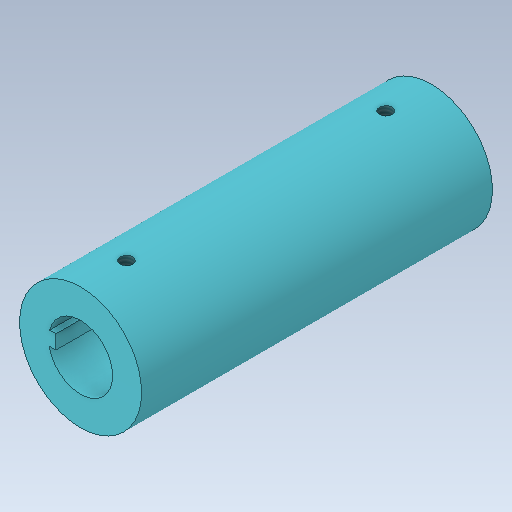
# Autodesk Inventor part: ShaftToConnectPotToMotor
Saved by Autodesk Inventor 2020.1 (Build 241239000, 239)
## iProperties
Created: 2018-02-27
Part Number: ShaftToConnectPotToMotor
Material: Aluminum 6061
Document SubType Name: Modeling
Designer: steele
Density: 2.7 g/cm^3
Appearance: Cadet Blue
Author: steele
Autodesk Inventor part; units mm, degrees
ref_plane "YZ Plane" through (0, 0, 0) normal (1, 0, 0) x (0, 1, 0)
ref_plane "XY Plane" through (0, 0, 0) normal (0, 0, 1) x (1, 0, 0)
sketch "Sketch2" plane through (0, 0, 0) normal (0, 0, 1) x (1, 0, 0)
  circle A0 centre (0, 0) radius 12.7
  dimension "d0" = 25.4
  constraints: 1 centre point, 1 coincident
  measures "d0" diameter of A0
extrude "Extrusion1" add sketch "Sketch2" along normal blind 73.025
sketch "Sketch3" plane through (0, 0, 73.025) normal (0, 0, 1) x (1, 0, 0)
  arc A0 (-6.5485, -1.2541) -> (-6.4558, 1.6669) centre (0, 0) ccw
  circle A1 centre (0, 0) radius 12.7 construction
  line L0 (-12.7, 0) -> (12.7, 0) construction
  line L1 (-6.35, 0) -> (-4.7625, 1.5875) construction
  line L2 (-4.7625, -1.5875) -> (-6.35, 0) construction
  line L3 (-6.5485, -1.2541) -> (-5.1223, -1.2541)
  line L4 (-5.1223, -1.2541) -> (-5.1223, 1.6669)
  line L5 (-5.1223, 1.6669) -> (-6.4558, 1.6669)
  dimension "d3" = 13.335
  dimension "d22" = 2.921
  dimension "d23" = 1.3335
  constraints: 12 end point, 4 point on circle, 2 horizontal, 2 perpendicular, 1 centre point, 1 coincident
  measures "d3" diameter of A0
  measures "d22" distance of L3.end L4.end
  measures "d23" distance of L4.end L5.end
extrude "Extrusion2" cut sketch "Sketch3" against normal blind 25.4
sketch "Sketch4" plane through (0, 0, 0) normal (0, 0, -1) x (-1, 0, 0)
  circle A0 centre (0, 0) radius 3.175
  dimension "d10" = 6.35
  constraints: 1 centre point, 1 coincident
  measures "d10" diameter of A0
extrude "Extrusion3" cut sketch "Sketch4" against normal through all
ref_plane "Work Plane1" through (0, 12.7, 0) normal (0, 1, 0) x (-1, 0, 0)
sketch "Sketch5" plane through (0, 12.7, 0) normal (0, 1, 0) x (-1, 0, 0)
  line L0 (-12.7, 0) -> (12.7, 0) projected
  point P0 (0, 0)
  point P1 (0, 9.525)
  dimension "d13" = 9.525
  measures "d13" distance from line of point (0, 9.525) L0
hole "Hole1" at (0, 12.7, 9.525) direction (0, -1, 0) diameter 2.6416 end through all thread size "6-32 UNC" class "2B" standard "ANSI Unified Screw Threads"
sketch "Sketch6" plane through (0, 12.7, 0) normal (0, 1, 0) x (-1, 0, 0)
  line L0 (12.7, 73.025) -> (-12.7, 73.025) projected
  point P0 (0, 0)
  point P1 (0, 63.5)
  dimension "d24" = 9.525
  measures "d24" distance from line of point (0, 63.5) L0
hole "Hole2" at (0, 12.7, 63.5) direction (0, -1, 0) diameter 2.6416 end through all thread size "6-32 UNC" class "2B" standard "ANSI Unified Screw Threads"
equation "\"d1\" = length"
equation "\"d3\" = shaftDiameter + shaftClearance"
equation "\"d22\" = keywayWidth"
equation "\"d23\" = keywayDepth"
equation "\"length\" = 73.025"
equation "\"shaftDiameter\" = 12.7"
equation "\"shaftClearance\" = 0.635"
equation "\"keywayWidth\" = 2.921"
equation "\"keywayDepth\" = 1.3335"
body "Solid1"
